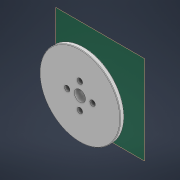
# Autodesk Inventor part: Pulley
Saved by Autodesk Inventor 2022 (Build 260153000, 153)
## iProperties
Created: 2022-01-13
Part Number: Pulley
Material: Generic
Document SubType Name: Modeling
Designer: izack
Density: 1 g/cm^3
Appearance: Default
Author: izack
Autodesk Inventor part; units mm, degrees
ref_plane "YZ Plane" through (0, 0, 0) normal (1, 0, 0) x (0, 1, 0)
ref_plane "XZ Plane" through (0, 0, 0) normal (0, 1, 0) x (-1, 0, 0)
ref_plane "XY Plane" through (0, 0, 0) normal (0, 0, 1) x (1, 0, 0)
sketch "Sketch1" plane through (0, 0, 0) normal (0, 1, 0) x (-1, 0, 0)
  line L0 (0, 0) -> (25.0825, 0)
  line L1 (25.0825, -25.4) -> (0, -25.4)
  line L2 (0, -25.4) -> (0, 0)
  line L3 (25.0825, -2.54) -> (11.8039, -2.54)
  line L4 (25.0825, -22.86) -> (11.8039, -22.86)
  line L5 (10.5339, -3.81) -> (10.5339, -21.59)
  line L6 (25.4, -0.3175) -> (25.4, -2.2225)
  line L7 (25.4, -23.1775) -> (25.4, -25.0825)
  arc A0 (25.4, -0.3175) -> (25.0825, 0) centre (25.0825, -0.3175) ccw
  arc A1 (25.0825, -2.54) -> (25.4, -2.2225) centre (25.0825, -2.2225) ccw
  arc A2 (25.4, -23.1775) -> (25.0825, -22.86) centre (25.0825, -23.1775) ccw
  arc A3 (25.0825, -25.4) -> (25.4, -25.0825) centre (25.0825, -25.0825) ccw
  arc A4 (11.8039, -2.54) -> (10.5339, -3.81) centre (11.8039, -3.81) ccw
  arc A5 (10.5339, -21.59) -> (11.8039, -22.86) centre (11.8039, -21.59) ccw
  point P0 (25.4, -25.4)
  point P1 (25.4, 0)
  dimension "d0" = 25.4
  dimension "d2" = 2.54
  dimension "d3" = 2.54
  dimension "d4" = 0.3175
  dimension "d5" = 1.27
  dimension "d7" = 25.4
  constraints: 16 end point, 12 point on circle, 12 tangent, 6 centre point, 4 equal radius, 4 point on line, 3 horizontal, 3 parallel, 2 perpendicular, 1 vertical
  measures "d0" distance of point (25.4, -25.4) L1.end
  measures "d2" distance between parallel lines of L0 L3
  measures "d3" distance between parallel lines of L1 L4
  measures "d4" radius of A0
  measures "d5" radius of A4
  measures "d7" distance of L1.end L0.start
revolve "Revolution1" add sketch "Sketch1" angle 360 about axis through (0, 0, -25.4) along (0, 0, 1)
sketch "Sketch2" plane through (0, 0, 0) normal (0, 0, 1) x (1, 0, 0)
  circle A0 centre (0, 0) radius 3.5
  circle A1 centre (0, 8) radius 1.7
  circle A2 centre (0, 0) radius 8
  circle A3 centre (-8, 0) radius 1.7
  circle A4 centre (0, -8) radius 1.7
  circle A5 centre (8, 0) radius 1.7
  dimension "d10" = 16
  dimension "d8" = 7
  dimension "d9" = 3.4
  dimension "d13" = 360
  constraints: 5 centre point, 2 coincident, 1 vertical alignment, 11 other
  measures "d8" diameter of A0
  measures "d9" diameter of A1
extrude "Extrusion1" cut sketch "Sketch2" against normal through all contours A0 | A1 A2 | A2 A1 | A3 A2 | A2 A3 | A5 A2 | A2 A5 | A4 A2 | A2 A4
ref_plane "Work Plane1" through (0, 0, -12.7) normal (0, 0, -1) x (-1, 0, 0)
sketch "Sketch3" plane through (0, 0, -25.4) normal (0, 0, -1) x (-1, 0, 0)
  circle A0 centre (0, 0) radius 25.4 projected
  point P0 (0, 0)
extrude "Extrusion2" cut sketch "Sketch3" against normal blind 12.7
body "Solid1"
